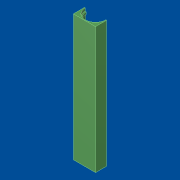
# Autodesk Inventor part: 402-gearbox-housing
Saved by Autodesk Inventor 2018 (Build 220112000, 112)
## iProperties
Created: 2020-06-11
Part Number: 402-gearbox-housing
Material: Generic
Document SubType Name: Modeling
Designer: Bunny320
Density: 1 g/cm^3
Appearance: Smooth - Dark Forest Green
Author: Bunny320
Autodesk Inventor part; units mm, degrees
ref_plane "YZ Plane" through (0, 0, 0) normal (1, 0, 0) x (0, 1, 0)
ref_plane "XZ Plane" through (0, 0, 0) normal (0, 1, 0) x (-1, 0, 0)
ref_plane "XY Plane" through (0, 0, 0) normal (0, 0, 1) x (1, 0, 0)
sketch "Sketch1" plane through (0, 0, 0) normal (0, 0, 1) x (1, 0, 0)
  line L0 (-19, -19) -> (19, -19)
  line L1 (19, -19) -> (19, 19)
  line L2 (19, 19) -> (-19, 19)
  line L3 (-19, 19) -> (-19, -19)
  line L4 (-19, -19) -> (19, 19) construction
  line L5 (19, -19) -> (-19, 19) construction
  point P0 (0, 0)
  dimension "d0" = 38
  constraints: 12 end point, 2 midpoint, 2 parallel, 2 perpendicular, 1 horizontal
  measures "d0" distance of L1.end L2.end
extrude "Extrusion1" add sketch "Sketch1" along normal blind 217
sketch "Sketch2" plane through (0, 0, 0) normal (0, 0, -1) x (-1, 0, 0)
  circle A0 centre (0, 0) radius 16.1
  dimension "d3" = 32.2
  constraints: 1 centre point, 1 coincident
  measures "d3" diameter of A0
extrude "Extrusion2" cut sketch "Sketch2" against normal blind 32
sketch "Sketch3" plane through (0, 0, 217) normal (0, 0, 1) x (1, 0, 0)
  circle A0 centre (0, 0) radius 17
  dimension "d6" = 34
  constraints: 1 centre point, 1 coincident
  measures "d6" diameter of A0
extrude "Extrusion3" cut sketch "Sketch3" against normal blind 177
sketch "Sketch4" plane through (0, 0, 40) normal (0, 0, 1) x (1, 0, 0)
  circle A0 centre (0, 0) radius 10
  dimension "d9" = 20
  constraints: 1 centre point, 1 coincident
  measures "d9" diameter of A0
extrude "Extrusion4" cut sketch "Sketch4" against normal through all
sketch "Sketch5" plane through (0, 0, 40) normal (0, 0, 1) x (1, 0, 0)
  point P0 (0, 0)
  point P1 (0, 13)
  dimension "d12" = 13
  constraints: 1 vertical alignment
  measures "d12" distance of point (0, 0) point (0, 13)
hole "Hole1" at (0, 13, 40) direction (0, 0, -1) diameter 3.4 end through all countersink diameter 7.5 countersink angle 90 clearance for "Countersunk Flat Head Hex Socket Screw DIN EN ISO 10642" size "M3" standard "DIN"
pattern_circular "Circular Pattern1" count 4 over 360 about axis through (0, 0, -10) along (0, 0, 1) of "Hole1"
sketch "Sketch7" plane through (0, 0, 0) normal (0, 1, 0) x (-1, 0, 0)
  line L0 (17, 80) -> (4.7, 80)
  line L1 (4.7, 80) -> (4.7, 83)
  line L2 (4.7, 83) -> (5, 83)
  line L3 (5, 83) -> (5, 86.1)
  line L4 (5, 86.1) -> (4.7, 86.1)
  line L5 (4.7, 86.1) -> (4.7, 89.1)
  line L6 (4.7, 89.1) -> (17, 89.1)
  line L7 (17, 217) -> (17, 40) projected
  line L8 (17, 89.1) -> (17, 80)
  line L9 (0, 88.2429) -> (0, 190.8877)
  line L10 (0, -42) -> (0, 252) projected
  line L11 (1.9638, 40) -> (9.8053, 40) projected
  line L12 (17, 167.9) -> (4.7, 167.9)
  line L13 (4.7, 167.9) -> (4.7, 170.9)
  line L14 (4.7, 170.9) -> (5, 170.9)
  line L15 (5, 170.9) -> (5, 174)
  line L16 (5, 174) -> (4.7, 174)
  line L17 (4.7, 174) -> (4.7, 177)
  line L18 (4.7, 177) -> (17, 177)
  line L19 (17, 177) -> (17, 167.9)
  line L20 (-17, 217) -> (17, 217) projected
  line L21 (17, 212) -> (16, 212)
  line L22 (16, 212) -> (16, 208)
  line L23 (16, 208) -> (17, 208)
  line L24 (17, 208) -> (17, 212)
  line L25 (17, 217) -> (17, 40) projected
  point P0 (0, 0)
  point P1 (1, 89.2429)
  dimension "d26" = 10
  dimension "d27" = 9.4
  dimension "d28" = 3.1
  dimension "d29" = 3
  dimension "d30" = 40
  dimension "d34" = 9.4
  dimension "d35" = 10
  dimension "d36" = 3
  dimension "d37" = 40
  dimension "d38" = 3.1
  dimension "d39" = 5
  dimension "d40" = 9
  dimension "d41" = 32
  constraints: 42 end point, 14 perpendicular, 8 point on line, 4 collinear, 3 horizontal, 1 vertical
  measures "d26" diameter of L3 L9
  measures "d27" diameter of L1 L9
  measures "d28" distance of L2.end L3.end
  measures "d29" distance of L4.end L5.end
  measures "d30" distance between parallel lines of L11 L0
  measures "d34" diameter of L13 L9
  measures "d35" diameter of L15 L9
  measures "d36" distance between parallel lines of L18 L16
  measures "d37" distance between parallel lines of L20 L18
  measures "d38" distance of L14.end L15.end
  measures "d39" distance between parallel lines of L20 L21
  measures "d40" distance between parallel lines of L20 L23
  measures "d41" diameter of L22 L9
revolve "Revolution1" add sketch "Sketch7" angle 360 about axis through (0, 0, 88.2429) along (0, 0, 1)
sketch "Sketch8" plane through (0, 0, 217) normal (0, 0, 1) x (1, 0, 0)
  circle A0 centre (0, 0) radius 17.75
  dimension "d42" = 35.5
  constraints: 1 centre point, 1 coincident
  measures "d42" diameter of A0
extrude "Extrusion6" cut sketch "Sketch8" against normal up to surface (5 mm away)
sketch "Sketch6" plane through (0, 0, 0) normal (0, 1, 0) x (-1, 0, 0)
  line L0 (-59.915, -50.2576) -> (49.2575, -50.2576)
  line L1 (49.2575, -50.2576) -> (49.2575, 450.4062)
  line L2 (49.2575, 450.4062) -> (-59.915, 450.4062)
  line L3 (-59.915, 450.4062) -> (-59.915, -50.2576)
  point P0 (0, 0)
  constraints: 8 end point, 2 parallel, 1 horizontal, 1 perpendicular
extrude "Extrusion5" cut sketch "Sketch6" along normal through all
equation "\"d34\" = d27"
equation "\"d35\" = d26"
equation "\"d36\" = d29"
equation "\"d37\" = d30"
equation "\"d38\" = d28"
body "Solid1"
